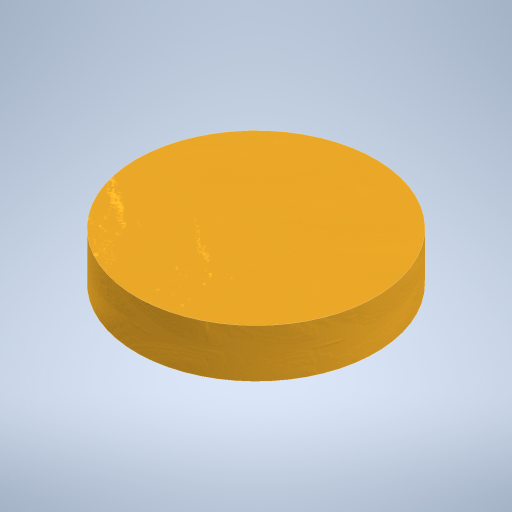
# Autodesk Inventor part: CapCenter
Saved by Autodesk Inventor 2024 (Build 280153000, 153)
## iProperties
Created: 2023-09-22
Part Number: CapCenter
Material: Brass, Soft Yellow, Welded
Document SubType Name: Modeling
Designer: schanen
Density: 8.5 g/cm^3
Appearance: Weld - Brass
Author: schanen
Autodesk Inventor part; units mm, degrees
ref_plane "YZ Plane" through (0, 0, 0) normal (1, 0, 0) x (0, 1, 0)
ref_plane "XZ Plane" through (0, 0, 0) normal (0, 1, 0) x (-1, 0, 0)
ref_plane "XY Plane" through (0, 0, 0) normal (0, 0, 1) x (1, 0, 0)
sketch "Sketch1" plane through (0, 0, 0) normal (0, 0, 1) x (1, 0, 0)
  line L0 (-19.225, -15) -> (-22.225, -15) construction
  line L1 (-22.225, -15) -> (-22.225, -5) construction
  line L2 (-22.225, -5) -> (-19.225, -5) construction
  line L3 (-19.225, -5) -> (-19.225, -15) construction
  line L4 (-20.225, 6) -> (-20.225, 0)
  line L5 (-22.225, 0) -> (-22.225, 9)
  line L6 (-22.225, 9) -> (0, 9)
  line L7 (0, 9) -> (0, 6)
  line L8 (0, 6) -> (-20.225, 6)
  line L9 (-19.225, -5) -> (-20.225, -5) construction
  line L10 (-20.225, -5) -> (-20.225, 0) construction
  line L11 (-20.225, 0) -> (-19.225, 0) construction
  line L12 (-19.225, 0) -> (-19.225, -5) construction
  line L13 (-22.225, 0) -> (-20.225, 0)
  point P0 (0, 0)
  point P1 (-19.225, 0)
  dimension "d0" = 10
  dimension "d1" = 22.225
  dimension "d3" = 3
  dimension "d16" = 3
  dimension "d17" = 1
  dimension "d18" = 5
  dimension "d19" = 6
  constraints: 28 end point, 4 horizontal, 4 horizontal alignment, 4 parallel, 4 perpendicular, 2 vertical, 2 vertical alignment, 1 coincident, 1 point on line
  measures "d0" distance of L0.end L1.end
  measures "d1" distance from line of point (0, 0) L1
  measures "d3" distance of L0.end L0.start
  measures "d16" distance of L6.end L7.end
  measures "d17" distance of L10.end L11.end
  measures "d18" distance of L9.end L10.end
  measures "d19" distance of L4.start L4.end
revolve "Revolution1" add sketch "Sketch1" angle 360 about axis through (0, 9, 0) along (0, -1, 0)
body "Solid1"
